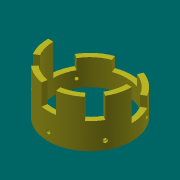
# Autodesk Inventor part: 知能ロボコン発射口
Saved by Autodesk Inventor 2013 (Build 170138000, 138)
## iProperties
Created: 2014-05-15
Part Number: 知能ロボコン発射口
Material: ABS プラスチック
Document SubType Name: Modeling
Designer: horumo136
Density: 1.06 g/cm^3
Mass: 63.0316 g
Surface Area: 287.494 cm^2
Volume: 59.4638 cm^3
Author: horumo136
Autodesk Inventor part; units mm, degrees
ref_plane "YZ Plane" through (0, 0, 0) normal (1, 0, 0) x (0, 1, 0)
ref_plane "XZ Plane" through (0, 0, 0) normal (0, 1, 0) x (-1, 0, 0)
sketch "スケッチ1" plane through (0, 0, 0) normal (0, 0, 1) x (1, 0, 0)
  line L0 (-45, -40) -> (45, -40)
  line L1 (45, -40) -> (45, 40)
  line L2 (45, 40) -> (-45, 40)
  line L3 (-45, 40) -> (-45, -40)
  line L4 (-45, -40) -> (45, 40) construction
  line L5 (45, -40) -> (-45, 40) construction
  point P0 (0, 0)
  dimension "d0" = 90
  dimension "d1" = 80
  constraints: 12 end point, 2 midpoint, 2 parallel, 1 horizontal, 1 perpendicular
  measures "d0" distance of L2.end L1.end
  measures "d1" distance of L1.end L0.end
extrude "押し出し1" add sketch "スケッチ1" along normal blind 5
sketch "スケッチ2" plane through (0, 0, 5) normal (0, 0, 1) x (1, 0, 0)
  circle A0 centre (0, 0) radius 40
  dimension "d4" = 80
  constraints: 1 centre point, 1 coincident
  measures "d4" diameter of A0
extrude "押し出し2" add sketch "スケッチ2" along normal blind 100
sketch "スケッチ3" plane through (0, 0, 105) normal (0, 0, 1) x (1, 0, 0)
  circle A0 centre (0, 0) radius 40 projected
  circle A1 centre (0, 0) radius 35
  dimension "d8" = 70
  constraints: 1 centre point, 1 coincident
  measures "d8" diameter of A1
extrude "押し出し3" cut sketch "スケッチ3" against normal blind 100 contours A1
sketch "スケッチ4" plane through (0, 0, 5) normal (0, 0, 1) x (1, 0, 0)
  circle A0 centre (0, 0) radius 35 projected
  circle A1 centre (0, 0) radius 27.5
  dimension "d11" = 55
  constraints: 1 centre point, 1 coincident
  measures "d11" diameter of A1
extrude "押し出し4" cut sketch "スケッチ4" against normal blind 5 contours A1
sketch "スケッチ5" plane through (0, 0, 105) normal (0, 0, 1) x (1, 0, 0)
  circle A0 centre (0, 0) radius 40 projected
  line L0 (-40, 0) -> (40, 0)
  constraints: 2 end point, 2 point on circle, 1 horizontal
extrude "押し出し5" cut sketch "スケッチ5" against normal blind 70 contours L0 A0 picked at (6.6667, 22.3933)
sketch "スケッチ6" plane through (0, 0, 105) normal (0, 0, 1) x (1, 0, 0)
  line L0 (-35, 0) -> (-40, 0) projected
  arc A0 (-40, 0) -> (40, 0) centre (0, 0) ccw projected
  line L1 (40, 0) -> (35, 0) projected
  arc A1 (-35, 0) -> (35, 0) centre (0, 0) ccw projected
extrude "押し出し6" cut sketch "スケッチ6" against normal blind 40
sketch "スケッチ7" plane through (0, 0, 65) normal (0, 0, 1) x (1, 0, 0)
  arc A0 (-40, 0) -> (40, 0) centre (0, 0) ccw projected
  arc A1 (-35, 0) -> (35, 0) centre (0, 0) ccw projected
  line L0 (0, 0) -> (6.9459, -39.3923)
  line L1 (0, 0) -> (40, 0) construction
  line L2 (0, 0) -> (-6.9459, -39.3923)
  arc A2 (-6.9459, -39.3923) -> (6.9459, -39.3923) centre (0, 0) ccw
  line L3 (0, 0) -> (-25.7115, -30.6418)
  line L4 (0, 0) -> (40, 0) construction
  line L5 (0, 0) -> (-34.641, -20)
  line L6 (0, 0) -> (40, 0) construction
  arc A3 (-34.641, -20) -> (-25.7115, -30.6418) centre (0, 0) ccw
  line L7 (0, 0) -> (40, 0) construction
  line L8 (0, 0) -> (16.9047, -36.2523)
  line L9 (0, 0) -> (40, 0) construction
  line L10 (0, 0) -> (25.7115, -30.6418)
  line L11 (0, 0) -> (34.641, -20)
  arc A4 (25.7115, -30.6418) -> (34.641, -20) centre (0, 0) ccw
  dimension "d18" = 80
  dimension "d19" = 130
  dimension "d20" = 150
  dimension "d22" = 65
  dimension "d23" = 30
  constraints: 24 end point, 11 point on circle, 5 horizontal, 4 equal length, 3 centre point, 2 symmetric about line, 1 concentric, 1 other
  measures "d18" angle of L0 L1
  measures "d19" angle of L3 L4
  measures "d20" angle of L5 L6
  measures "d22" angle of L8 L9
  measures "d23" angle of L2 L3
extrude "押し出し7" cut sketch "スケッチ7" against normal blind 40 contours L5 A1 L3 A0 | L5 L3 A1 | L2 A1 L0 A0 | L0 A1 L2 | L11 A1 L10 | A1 L11 A0 L10
sketch "スケッチ8" plane through (0, 0, 35) normal (0, 0, 1) x (1, 0, 0)
  arc A0 (40, 0) -> (-40, 0) centre (0, 0) ccw projected
  line L0 (0, 0) -> (-13.6808, 37.5877)
  line L1 (0, 0) -> (40, 0) construction
  line L2 (0, 0) -> (13.6808, 37.5877)
  arc A1 (13.6808, 37.5877) -> (-13.6808, 37.5877) centre (0, 0) ccw
  line L3 (0, 0) -> (40, 0)
  line L4 (0, 0) -> (40, 0) construction
  arc A2 (40, 0) -> (34.641, 20) centre (0, 0) ccw
  line L5 (0, 0) -> (-40, 0)
  line L6 (0, 0) -> (-34.641, 20)
  line L7 (0, 0) -> (40, 0) construction
  arc A3 (-34.641, 20) -> (-40, 0) centre (0, 0) ccw
  line L8 (0, 0) -> (0, 40)
  arc A4 (40, 0) -> (-40, 0) centre (0, 0) ccw
  line L9 (0, 0) -> (40, 0)
  line L10 (0, 0) -> (34.641, 20)
  dimension "d26" = 110
  dimension "d28" = 150
  constraints: 22 end point, 13 point on circle, 4 centre point, 3 horizontal, 2 collinear, 2 concentric, 2 equal length, 2 symmetric about line, 1 other
  measures "d26" angle of L1 L0
  measures "d28" angle of L7 L6
extrude "押し出し8" cut sketch "スケッチ8" against normal blind 30 contours L8 A0 L2 | L5 A0 L6 | L0 A0 L8
sketch "スケッチ9" plane through (0, 0, 35) normal (0, 0, 1) x (1, 0, 0)
  line L0 (40, 0) -> (35, 0) projected
  arc A0 (40, 0) -> (13.6808, 37.5877) centre (0, 0) ccw projected
  line L1 (0, 0) -> (40, 0)
  line L2 (0, 0) -> (34.641, 20)
  line L3 (0, 0) -> (40, 0) construction
  arc A1 (40, 0) -> (34.641, 20) centre (0, 0) ccw
  dimension "d31" = 30
  constraints: 6 end point, 3 point on circle, 1 centre point, 1 collinear, 1 concentric, 1 equal length, 1 horizontal
  measures "d31" angle of L3 L2
extrude "押し出し9" cut sketch "スケッチ9" against normal blind 30
sketch "スケッチ10" plane through (0, 0, 0) normal (0, 0, -1) x (-1, 0, 0)
  line L0 (-45, 40) -> (-35, 40)
  line L1 (-35, 40) -> (-35, 30)
  line L2 (-35, 30) -> (-45, 30)
  line L3 (-45, 30) -> (-45, 40)
  line L4 (-45, -40) -> (-35, -40)
  line L5 (-35, -40) -> (-35, -30)
  line L6 (-35, -30) -> (-45, -30)
  line L7 (-45, -30) -> (-45, -40)
  line L8 (45, -40) -> (35, -40)
  line L9 (35, -40) -> (35, -30)
  line L10 (35, -30) -> (45, -30)
  line L11 (45, -30) -> (45, -40)
  line L12 (45, 40) -> (35, 40)
  line L13 (35, 40) -> (35, 30)
  line L14 (35, 30) -> (45, 30)
  line L15 (45, 30) -> (45, 40)
  dimension "d34" = 10
  dimension "d35" = 10
  dimension "d36" = 10
  dimension "d37" = 10
  dimension "d38" = 10
  dimension "d39" = 10
  dimension "d40" = 10
  dimension "d41" = 10
  constraints: 32 end point, 8 parallel, 4 coincident, 4 horizontal, 4 perpendicular
  measures "d34" distance of L1.end L2.end
  measures "d35" distance of L0.end L1.end
  measures "d36" distance of L6.end L5.end
  measures "d37" distance of L5.end L4.end
  measures "d38" distance of L9.end L10.end
  measures "d39" distance of L8.end L9.end
  measures "d40" distance of L14.end L13.end
  measures "d41" distance of L13.end L12.end
hole "穴1" at (35, -30, 0) at (-35, -30, 0) at (-35, 30, 0) at (35, 30, 0) direction (0, 0, 1) diameter 3 depth 8 tip angle 118
sketch "スケッチ11" plane through (0, 0, 5) normal (0, 0, 1) x (1, 0, 0)
  circle A0 centre (-35, 30) radius 1.5 projected
  circle A1 centre (35, -30) radius 1.5 projected
  circle A2 centre (-35, -30) radius 1.5 projected
  circle A3 centre (35, 30) radius 1.5 projected
  line L0 (0, -40) -> (45, -40) projected
  line L1 (45, -40) -> (45, 40) projected
  line L2 (45, 40) -> (-45, 40) projected
  line L3 (-45, 40) -> (-45, -40) projected
  line L4 (-45, -40) -> (0, -40) projected
  circle A4 centre (0, 0) radius 27.5 projected
  circle A5 centre (0, 0) radius 40
  dimension "d49" = 80
  constraints: 1 centre point, 1 coincident
  measures "d49" diameter of A5
extrude "押し出し10" cut sketch "スケッチ11" against normal blind 10 contours A5 L2 L1 L0 | L4 L3 L2 A5
sketch "スケッチ12" plane through (0, 0, 5) normal (0, 0, 1) x (1, 0, 0)
  arc A0 (-34.641, 20) -> (-40, 0) centre (0, 0) ccw projected
  line L0 (-35, 0) -> (-40, 0) projected
  arc A1 (-35, 0) -> (35, 0) centre (0, 0) ccw projected
  line L1 (40, 0) -> (35, 0) projected
  arc A2 (40, 0) -> (34.641, 20) centre (0, 0) ccw projected
  line L2 (30.3109, 17.5) -> (34.641, 20) projected
  arc A3 (30.3109, 17.5) -> (11.9707, 32.8892) centre (0, 0) ccw projected
  line L3 (13.6808, 37.5877) -> (11.9707, 32.8892) projected
  arc A4 (13.6808, 37.5877) -> (-13.6808, 37.5877) centre (0, 0) ccw projected
  line L4 (-11.9707, 32.8892) -> (-13.6808, 37.5877) projected
  arc A5 (-11.9707, 32.8892) -> (-30.3109, 17.5) centre (0, 0) ccw projected
  line L5 (-34.641, 20) -> (-30.3109, 17.5) projected
  circle A6 centre (0, 0) radius 35
  circle A7 centre (0, 0) radius 40
  dimension "d52" = 80
  constraints: 2 centre point, 2 coincident, 1 concentric
  measures "d52" diameter of A7
extrude "押し出し11" add sketch "スケッチ12" along normal blind 10 contours L5 A6 L0 A0 | A4 L3 A6 L4 | L1 A6 L2 A2
ref_plane "作業平面1" through (0, 40, 15) normal (0, 1, 0) x (-1, 0, 0)
sketch "スケッチ13" plane through (0, 40, 15) normal (0, 1, 0) x (-1, 0, 0)
  line L0 (0, -15) -> (0, -7)
  dimension "d55" = 8
  constraints: 2 end point, 1 coincident, 1 vertical
  measures "d55" distance of L0.start L0.end
hole "穴2" at (0, 40, 8) direction (0, -1, 0) diameter 3 depth 8 tip angle 118 counterbore diameter 4 counterbore depth 2
pattern_circular "円形状パターン1" count 6 over 360 about axis through (0, 0, 105) along (0, 0, -1) of "穴2"
sketch "スケッチ14" plane through (0, 0, 5) normal (0, 0, 1) x (1, 0, 0)
  circle A0 centre (0, 0) radius 35 projected
  circle A1 centre (0, 0) radius 27.5 projected
extrude "押し出し12" cut sketch "スケッチ14" against normal blind 10
sketch "スケッチ15" plane through (0, 0, 35) normal (0, 0, 1) x (1, 0, 0)
  line L0 (-11.9707, 32.8892) -> (-13.6808, 37.5877) projected
  arc A0 (-13.6808, 37.5877) -> (-34.641, 20) centre (0, 0) ccw projected
  line L1 (-34.641, 20) -> (-30.3109, 17.5) projected
  arc A1 (-11.9707, 32.8892) -> (-30.3109, 17.5) centre (0, 0) ccw projected
  line L2 (-40.9494, 9.0736) -> (38.994, 9.0736)
  line L3 (38.994, 9.0736) -> (38.994, 41.7368)
  line L4 (38.994, 41.7368) -> (-40.9494, 41.7368)
  line L5 (-40.9494, 41.7368) -> (-40.9494, 9.0736)
  constraints: 8 end point, 2 parallel, 1 horizontal, 1 perpendicular
extrude "押し出し13" cut sketch "スケッチ15" against normal blind 10 contours A1 L1 A0 L0 | L5 L4 L3 L2
sketch "スケッチ16" plane through (0, 0, 65) normal (0, 0, 1) x (1, 0, 0)
  line L0 (25.7115, -30.6418) -> (22.4976, -26.8116) projected
  arc A0 (6.0777, -34.4683) -> (22.4976, -26.8116) centre (0, 0) ccw projected
  line L1 (6.0777, -34.4683) -> (6.9459, -39.3923) projected
  arc A1 (6.9459, -39.3923) -> (25.7115, -30.6418) centre (0, 0) ccw projected
  line L2 (41.1854, 0) -> (-41.2126, 0)
  line L3 (-41.2126, 0) -> (-41.2126, -41.1487)
  line L4 (-41.2126, -41.1487) -> (41.1854, -41.1487)
  line L5 (41.1854, -41.1487) -> (41.1854, 0)
  constraints: 8 end point, 2 parallel, 1 horizontal, 1 perpendicular
extrude "押し出し14" cut sketch "スケッチ16" against normal blind 20 contours A1 L1 A0 L0 | L5 L4 L3 L2
